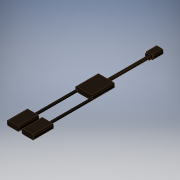
# Autodesk Inventor part: phone wire
Saved by Autodesk Inventor 2017 (Build 210142000, 142)
## iProperties
Created: 2017-12-02
Part Number: phone wire
Material: PAEK Plastic
Document SubType Name: Modeling
Designer: User
Density: 1.32 g/cm^3
Appearance: Smooth - White
Author: User
Autodesk Inventor part; units mm, degrees
ref_plane "YZ Plane" through (0, 0, 0) normal (1, 0, 0) x (0, 1, 0)
ref_plane "XZ Plane" through (0, 0, 0) normal (0, 1, 0) x (-1, 0, 0)
ref_plane "XY Plane" through (0, 0, 0) normal (0, 0, 1) x (1, 0, 0)
sketch "Sketch1" plane through (0, 0, 0) normal (0, 1, 0) x (-1, 0, 0)
  line L0 (0, 0) -> (9.525, 0)
  line L1 (9.525, 0) -> (9.525, -12.7)
  line L2 (9.525, -12.7) -> (0, -12.7)
  line L3 (0, -12.7) -> (0, 0)
  line L4 (7.9375, 0) -> (1.5875, 0)
  line L5 (1.5875, 0) -> (1.5875, 2.7348)
  line L6 (1.5875, 2.7348) -> (7.9375, 2.7348)
  line L7 (7.9375, 2.7348) -> (7.9375, 0)
  line L8 (6.35, 2.7348) -> (3.175, 2.7348)
  line L9 (3.175, 2.7348) -> (3.175, 56.7098)
  line L10 (3.175, 56.7098) -> (6.35, 56.7098)
  line L11 (6.35, 56.7098) -> (6.35, 2.7348)
  line L12 (15.875, 56.7098) -> (-6.35, 56.7098)
  line L13 (-6.35, 56.7098) -> (-6.35, 85.2848)
  line L14 (-6.35, 85.2848) -> (15.875, 85.2848)
  line L15 (15.875, 85.2848) -> (15.875, 56.7098)
  line L16 (15.875, 85.2848) -> (12.7, 85.2848)
  line L17 (12.7, 85.2848) -> (12.7, 142.4348)
  line L18 (12.7, 142.4348) -> (15.875, 142.4348)
  line L19 (15.875, 142.4348) -> (15.875, 85.2848)
  line L20 (-6.35, 85.2848) -> (-3.175, 85.2848)
  line L21 (-3.175, 85.2848) -> (-3.175, 142.4348)
  line L22 (-3.175, 142.4348) -> (-6.35, 142.4348)
  line L23 (-6.35, 142.4348) -> (-6.35, 85.2848)
  line L24 (6.35, 142.4348) -> (22.225, 142.4348)
  line L25 (22.225, 142.4348) -> (22.225, 167.8348)
  line L26 (22.225, 167.8348) -> (6.35, 167.8348)
  line L27 (6.35, 167.8348) -> (6.35, 142.4348)
  line L28 (-12.7, 142.4348) -> (3.175, 142.4348)
  line L29 (3.175, 142.4348) -> (3.175, 167.8348)
  line L30 (3.175, 167.8348) -> (-12.7, 167.8348)
  line L31 (-12.7, 167.8348) -> (-12.7, 142.4348)
  dimension "d0" = 9.525
  dimension "d1" = 12.7
  dimension "d2" = 6.35
  dimension "d3" = 3.175
  dimension "d4" = 53.975
  dimension "d5" = 1.5875
  dimension "d6" = 3.175
  dimension "d7" = 1.5875
  dimension "d8" = 1.5875
  dimension "d9" = 22.225
  dimension "d10" = 28.575
  dimension "d11" = 9.525
  dimension "d12" = 53.975
  dimension "d13" = 28.575
  dimension "d14" = 2.7348
  dimension "d15" = 3.175
  dimension "d16" = 3.175
  dimension "d17" = 57.15
  dimension "d18" = 15.875
  dimension "d19" = 25.4
  dimension "d20" = 6.35
  dimension "d21" = 57.15
  dimension "d22" = 15.875
  dimension "d23" = 25.4
  dimension "d24" = 57.15
  dimension "d25" = 6.35
  constraints: 64 end point, 16 parallel, 8 horizontal, 8 perpendicular, 4 point on line
  measures "d0" distance of L1.end L2.end
  measures "d1" distance of L0.end L1.end
  measures "d2" distance of L5.end L6.end
  measures "d3" distance of L9.end L10.end
  measures "d4" distance of L8.end L9.end
  measures "d5" distance of L6.end L8.start
  measures "d6" distance between parallel lines of L9 L11
  measures "d7" distance between parallel lines of L1 L7
  measures "d8" distance from line of L11 L6.end
  measures "d9" distance of L13.end L14.end
  measures "d10" distance between parallel lines of L14 L10
  measures "d11" distance between parallel lines of L11 L15
  measures "d12" distance between parallel lines of L6 L12
  measures "d13" distance between parallel lines of L12 L14
  measures "d14" distance between parallel lines of L0 L6
  measures "d15" distance of L17.end L18.end
  measures "d16" distance between parallel lines of L23 L21
  measures "d17" distance between parallel lines of L20 L22
  measures "d18" distance of L26.end L25.end
  measures "d19" distance of L25.end L24.end
  measures "d20" distance between parallel lines of L19 L25
  measures "d21" distance between parallel lines of L14 L24
  measures "d22" distance between parallel lines of L31 L29
  measures "d23" distance between parallel lines of L28 L30
  measures "d24" distance between parallel lines of L14 L28
  measures "d25" distance between parallel lines of L21 L29
extrude "Extrusion1" add sketch "Sketch1" along normal blind 6.35 contours L0 L1 L2 L3
extrude "Extrusion2" add sketch "Sketch1" along normal blind 6.35 contours L5 L6 L7 L0
extrude "Extrusion3" add sketch "Sketch1" along normal blind 3.175 contours L9 L10 L11 L6
extrude "Extrusion4" add sketch "Sketch1" along normal blind 6.35 contours L12 L13 L14 L15 L10
extrude "Extrusion5" add sketch "Sketch1" along normal blind 3.175 contours L23 L22 L21 L14 | L14 L17 L18 L19
extrude "Extrusion6" add sketch "Sketch1" along normal blind 6.35 contours L28 L31 L30 L29 L22 | L18 L24 L27 L26 L25
fillet "Fillet1" radius 1.5875 28 edges at (-22.225, 6.35, 155.1348) (-6.35, 6.35, 155.1348) (-12.7, 3.175, 113.8598) (-15.875, 3.175, 113.8598) (-15.875, 0, 99.5723) (-12.7, 0, 113.8598) (3.175, 0, 113.8598) (6.35, 0, 99.5723) (6.35, 6.35, 70.9973) (-3.175, 0, 29.7223) (-6.35, 0, 29.7223) (0, 0, -6.35) (-9.525, 0, -6.35) (-1.5875, 0, 1.3674) (-7.9375, 0, 1.3674) (12.7, 0, 155.1348) (-3.175, 0, 155.1348) (0, 6.35, -6.35) (-9.525, 6.35, -6.35) (-15.875, 6.35, 70.9973) (-3.175, 6.35, 155.1348) (12.7, 6.35, 155.1348) (-6.35, 0, 155.1348) (-22.225, 0, 155.1348) (-7.9375, 6.35, 1.3674) (-1.5875, 6.35, 1.3674) (3.175, 3.175, 113.8598) (6.35, 3.175, 113.8598)
equation "\"d5\" = 0.5 * d6"
equation "\"d22\" = d18"
equation "\"d23\" = d19"
body "Solid1"
